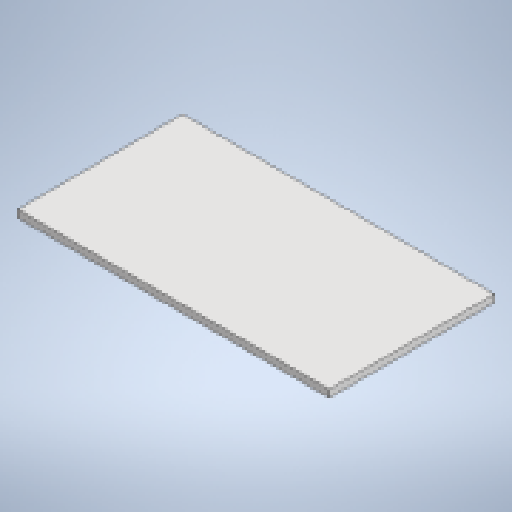
# Autodesk Inventor part: BASE
Saved by Autodesk Inventor 2025.1 (Build 291241000, 241)
## iProperties
Created: 2025-05-08
Part Number: BASE
Material: Generic
Document SubType Name: Modeling
Designer: User
Density: 1 g/cm^3
Appearance: Default
Author: User
Autodesk Inventor part; units mm, degrees
ref_plane "YZ Plane" through (0, 0, 0) normal (1, 0, 0) x (0, 1, 0)
sketch "Sketch1" plane through (0, 0, 0) normal (0, 1, 0) x (-1, 0, 0)
  line L0 (61.5114, -24.7991) -> (-86.6751, -24.7991)
  line L1 (-86.6751, -24.7991) -> (-86.6751, 53.6097)
  line L2 (-86.6751, 53.6097) -> (61.5114, 53.6097)
  line L3 (61.5114, 53.6097) -> (61.5114, -24.7991)
  point P0 (0, 0)
  constraints: 8 end point, 2 parallel, 1 horizontal, 1 perpendicular
extrude "Extrusion1" add sketch "Sketch1" along normal blind 3.5
sketch "Sketch2" plane through (-61.5114, 0, -24.7991) normal (-1, 0, 0) x (0, 0, 1)
  line L0 (0, 0) -> (78.4088, 0) projected
  line L1 (78.4088, 0) -> (78.4088, 3.5) projected
  line L2 (0, 3.5) -> (78.4088, 3.5) projected
  line L3 (0, 0) -> (0, 3.5) projected
  point P0 (24.7991, 0)
ref_plane "Work Plane1" through (46.6751, -27, 13.6097) normal (-1, 0, 0) x (0, 0, 1)
extrude "Extrusion2" cut sketch "Sketch2" against normal up to surface (108.1865 mm away)
sketch "Sketch3" plane through (86.6751, 0, -24.7991) normal (0, 0, -1) x (-1, 0, 0)
  line L0 (40, 0) -> (40, 3.5) projected
  line L1 (0, 3.5) -> (40, 3.5) projected
  line L2 (0, 0) -> (0, 3.5) projected
  line L3 (0, 0) -> (40, 0) projected
  point P0 (86.6751, 0)
ref_plane "Work Plane2" through (49.1751, -3, 11.1097) normal (0, 0, -1) x (0, 1, 0)
extrude "Extrusion3" cut sketch "Sketch3" against normal up to surface (35.9088 mm away)
sketch "Sketch4" plane through (0, 3.5, 0) normal (0, 1, 0) x (1, 0, 0)
  line L0 (46.6751, -53.6097) -> (86.6751, -53.6097) projected
  point P0 (0, 0)
body "Solid1"
